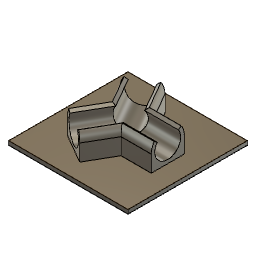
3servojoint v1 (Autodesk Fusion 360 design; units mm, degrees)
Autodesk Fusion 360 part; units mm, degrees
sketch "スケッチ1" plane through (0, 0, 0) normal (0, 1, 0) x (1, 0, 0)
  line L0 (15, -15) -> (-15, -15)
  line L1 (-15, -15) -> (-15, 15)
  line L2 (-15, 15) -> (15, 15)
  line L3 (15, 15) -> (15, -15)
  line L4 (15, -15) -> (-15, 15) construction
  line L5 (-15, -15) -> (15, 15) construction
  dimension "d1" = 30
  dimension "d2" = 30
  constraint perpendicular L0 L1
  constraint parallel L0 L2
  constraint parallel L1 L3
  constraint horizontal L0
  constraint coincident L4 origin
  constraint coincident L5 origin
  measures "d1" distance of L1.end L2.end
  measures "d2" distance of L0.end L1.end
sketch "スケッチ2" plane through (0, 0, 0) normal (1, 0, 0) x (0, 0, -1)
extrude "押し出し1" add sketch "スケッチ1" along normal blind 1 makes body 1
sketch "スケッチ3" plane through (0, 1, 0) normal (0, 1, 0) x (-1, 0, 0)
  line L0 (-15, -15) -> (15, -15)
  line L1 (15, -15) -> (15, 15)
  line L2 (15, 15) -> (-15, 15)
  line L3 (-15, 15) -> (-15, -15)
sketch "スケッチ4" plane through (0, 0, 0) normal (1, 0, 0) x (0, 0, -1)
  line L0 (0, 1) -> (0, 9.3)
  circle A0 centre (0, 5.15) radius 4.15
  circle A1 centre (0, 5.15) radius 3.25
  line L1 (0, 1) -> (-4.15, 1)
  line L2 (-4.15, 1) -> (-4.15, 5.15)
  line L3 (0, 1) -> (4.15, 1)
  line L4 (4.15, 1) -> (4.15, 5.15)
  line L5 (0, 5.15) -> (3.3995, 7.5303)
  line L6 (0, 5.15) -> (4.15, 5.15) construction
  line L7 (0, 5.15) -> (-3.3995, 7.5303)
  line L8 (0, 5.15) -> (4.15, 5.15) construction
  point P0 (0, 1)
  dimension "d5" = 8.3
  dimension "d6" = 6.5
  dimension "d7" = 4.15
  dimension "d16" = 35
  dimension "d17" = 145
  constraint coincident P0 L0.start
  constraint vertical L0
  constraint midpoint L0 A0.centre
  constraint coincident L0.end A0
  constraint concentric A0 A1
  constraint perpendicular L0 L1
  constraint coincident A0 L2.end
  constraint tangent A0 L2
  constraint symmetric P0 L0 L1.start
  constraint symmetric L0 L1.end L3.end
  constraint symmetric L0 L2.end L4.end
  constraint horizontal L6
  constraint coincident A0.centre A1.centre
  constraint horizontal L8
  measures "d5" distance of P0 L0.end
  measures "d6" diameter of A1
  measures "d7" distance of P0 L1.end
  measures "d16" angle of L5 L6
  measures "d17" angle of L7 L8
extrude "押し出し2" add sketch "スケッチ4" along normal blind 10 separate body contours L0 A0 A1 L7 | A0 L1 L2 | L0 A0 A1 L5 | A0 L3 L4 picked at (-3.8286, 4.8274) picked at (3.8249, 4.799) makes body 2
pattern_circular "C パターン1" count 3 over 360 about axis through (0, 1.75, 0) along (0, 1, 0) of bodies 2 makes body 3 at (-0.7077, 6.3206, -7.2894) makes body 4 at (-6.1395, 5.4019, 4.1534)
ref_plane "作業平面1" through (-2.5, 3.075, 4.3301) normal (0.866025, 0, 0.5) x (0, 1, 0)
sketch "スケッチ5" plane through (-2, 2.375, 3.4641) normal (0.866025, 0, 0.5) x (0, 1, 0)
ref_plane "作業平面2" through (-2.5, 3.075, -4.3301) normal (0.866025, 0, -0.5) x (0, -1, 0)
ref_plane "作業平面3" through (-2.5, 3.075, 4.3301) normal (0.866025, 0, 0.5) x (0, 1, 0)
split "分割1" by plane through (-2.5, 3.075, -4.3301) normal (0.866025, 0, -0.5) bodies 2 makes body 5 at (6.7079, 1.9081, 0.2289)
split "分割2" by plane through (-2.5, 3.075, 4.3301) normal (0.866025, 0, 0.5) bodies 5 makes body 6 at (6.7079, 1.9081, 0.2289)
pattern_circular "C パターン2" count 3 over 360 about axis through (0, 1.75, 0) along (0, 1, 0) of bodies 6 makes body 7 at (-3.1284, 1.9118, -5.971) makes body 8 at (-3.6069, 1.9118, 5.6948)
hidden bodies 2 3 4 5
